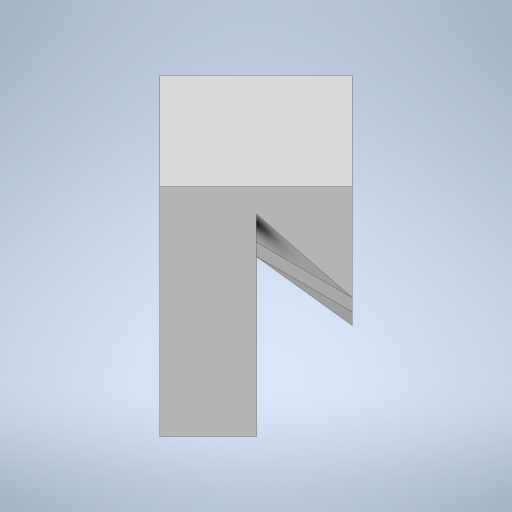
# Autodesk Inventor part: Деталь1
Saved by Autodesk Inventor 2023.2 (Build 272271030, 271C)
## iProperties
Created: 2023-09-29
Part Number: Деталь1
Material: Типовые
Document SubType Name: Modeling
Designer: User
Density: 1 g/cm^3
Appearance: По умолчанию
Author: User
Autodesk Inventor part; units mm, degrees
ref_plane "YZ Plane" through (0, 0, 0) normal (1, 0, 0) x (0, 1, 0)
ref_plane "XZ Plane" through (0, 0, 0) normal (0, 1, 0) x (-1, 0, 0)
ref_plane "XY Plane" through (0, 0, 0) normal (0, 0, 1) x (1, 0, 0)
sketch "Эскиз4" plane through (0, 0, 0) normal (0, 1, 0) x (-1, 0, 0)
  line L0 (-40, 0) -> (0, 40)
  line L1 (0, 40) -> (40, 0)
  line L2 (40, 0) -> (0, -40)
  line L3 (0, -40) -> (-40, 0)
  point P0 (0, 0)
  point P1 (0, 0)
  constraints: 8 end point, 9 other
extrude "Выдавливание2" add sketch "Эскиз4" along normal blind 90
sketch "Эскиз5" plane through (0, 0, 0) normal (1, 0, 0) x (0, 1, 0)
  line L0 (50, -19.8959) -> (-50, -19.8959)
  line L1 (-50, -19.8959) -> (-50, 19.8959)
  line L2 (-50, 19.8959) -> (50, 19.8959)
  line L3 (50, 19.8959) -> (50, -19.8959)
  line L4 (0, 0) -> (0, 40) projected
  line L5 (50, -19.8959) -> (-50, 19.8959) construction
  line L6 (-50, -19.8959) -> (50, 19.8959) construction
  line L7 (0, -40) -> (0, 0) projected
  line L8 (0, -40) -> (25, -19.8959)
  line L9 (0, 0) -> (90, 0) projected
  line L10 (50, 0) -> (80, 19.8959)
  line L11 (80, 19.8959) -> (50, 19.8959)
  line L12 (90, 0) -> (90, 40) projected
  point P0 (90, 20)
  point P1 (0, 19.8959)
  dimension "d8" = 100
  dimension "d9" = 25
  dimension "d10" = 10
  constraints: 18 end point, 4 midpoint, 2 horizontal, 2 parallel, 2 point on line, 1 perpendicular
  measures "d8" distance of L1.end L2.end
  measures "d9" horizontal distance of L7.start L8.end
  measures "d10" horizontal distance of point (90, 20) L10.end
extrude "Выдавливание3" cut sketch "Эскиз5" along normal mid plane 150 contours L0 L7 L9 L3 | L8 L7 L0 | L9 L4 L2 L3 | L3 L11 L10
